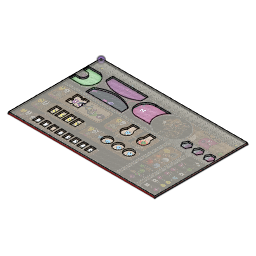
Gaia Project (Autodesk Fusion 360 design; units mm, degrees)
Autodesk Fusion 360 part; units mm, degrees
sketch "Sketch1" plane through (0, 0, 0) normal (0, 1, 0) x (1, 0, 0)
  line L0 (0, 0) -> (300, 0)
  line L1 (300, 0) -> (300, -190)
  line L2 (300, -190) -> (0, -190)
  line L3 (0, -190) -> (0, 0)
  dimension "d1" = 300
  dimension "d2" = 190
  constraint horizontal L0
  constraint vertical L1
  constraint horizontal L2
  constraint vertical L3
  constraint coincident L0.start L3.end
  measures "d1" distance of L0.start L0.end
  measures "d2" distance of L0.start L2.end
sketch "Sketch2" plane through (0, 0, 0) normal (0, 1, 0) x (1, 0, 0)
  line L0 (0, 0) -> (300, 0)
  line L1 (300, 0) -> (300, -190)
  line L2 (300, -190) -> (0, -190)
  line L3 (0, -190) -> (0, 0)
  line L4 (38.8424, -166.0412) -> (48.8424, -166.0412)
  line L5 (48.8424, -166.0412) -> (48.8424, -180.0412)
  line L6 (48.8424, -180.0412) -> (38.8424, -180.0412)
  line L7 (38.8424, -180.0412) -> (38.8424, -166.0412)
  line L8 (64.0567, -180.0412) -> (54.0567, -180.0412)
  line L9 (54.0567, -180.0412) -> (54.0567, -166.0412)
  line L10 (54.0567, -166.0412) -> (64.0567, -166.0412)
  line L11 (64.0567, -166.0412) -> (64.0567, -180.0412)
  line L12 (79.271, -180.0412) -> (69.271, -180.0412)
  line L13 (69.271, -180.0412) -> (69.271, -166.0412)
  line L14 (69.271, -166.0412) -> (79.271, -166.0412)
  line L15 (79.271, -166.0412) -> (79.271, -180.0412)
  line L16 (94.4853, -180.0412) -> (84.4853, -180.0412)
  line L17 (84.4853, -180.0412) -> (84.4853, -166.0412)
  line L18 (84.4853, -166.0412) -> (94.4853, -166.0412)
  line L19 (94.4853, -166.0412) -> (94.4853, -180.0412)
  line L20 (109.6995, -180.0412) -> (99.6995, -180.0412)
  line L21 (99.6995, -180.0412) -> (99.6995, -166.0412)
  line L22 (99.6995, -166.0412) -> (109.6995, -166.0412)
  line L23 (109.6995, -166.0412) -> (109.6995, -180.0412)
  line L24 (124.9138, -180.0412) -> (114.9138, -180.0412)
  line L25 (114.9138, -180.0412) -> (114.9138, -166.0412)
  line L26 (114.9138, -166.0412) -> (124.9138, -166.0412)
  line L27 (124.9138, -166.0412) -> (124.9138, -180.0412)
  line L28 (140.1281, -180.0412) -> (130.1281, -180.0412)
  line L29 (130.1281, -180.0412) -> (130.1281, -166.0412)
  line L30 (130.1281, -166.0412) -> (140.1281, -166.0412)
  line L31 (140.1281, -166.0412) -> (140.1281, -180.0412)
  line L32 (155.3424, -180.0412) -> (145.3424, -180.0412)
  line L33 (145.3424, -180.0412) -> (145.3424, -166.0412)
  line L34 (145.3424, -166.0412) -> (155.3424, -166.0412)
  line L35 (155.3424, -166.0412) -> (155.3424, -180.0412)
  line L36 (38.4602, -129.9646) -> (49.4602, -129.9646)
  line L37 (49.4602, -129.9646) -> (49.4602, -148.9646)
  line L38 (49.4602, -148.9646) -> (38.4602, -148.9646)
  line L39 (38.4602, -148.9646) -> (38.4602, -129.9646)
  line L40 (53.6269, -129.9646) -> (64.6269, -129.9646)
  line L41 (64.6269, -129.9646) -> (64.6269, -148.9646)
  line L42 (64.6269, -148.9646) -> (53.6269, -148.9646)
  line L43 (53.6269, -148.9646) -> (53.6269, -129.9646)
  line L44 (68.7936, -129.9646) -> (79.7936, -129.9646)
  line L45 (79.7936, -129.9646) -> (79.7936, -148.9646)
  line L46 (79.7936, -148.9646) -> (68.7936, -148.9646)
  line L47 (68.7936, -148.9646) -> (68.7936, -129.9646)
  line L48 (83.9602, -129.9646) -> (94.9602, -129.9646)
  line L49 (94.9602, -129.9646) -> (94.9602, -148.9646)
  line L50 (94.9602, -148.9646) -> (83.9602, -148.9646)
  line L51 (83.9602, -148.9646) -> (83.9602, -129.9646)
  circle A0 centre (151.5176, -138.9113) radius 9.55
  circle A1 centre (173.7676, -138.9113) radius 9.55
  circle A2 centre (196.0176, -138.9113) radius 9.55
  line L52 (163.1466, -84.6487) -> (163.1466, -96.6053)
  line L53 (150.1466, -96.8262) -> (150.1466, -84.6487)
  arc A3 (150.1466, -96.8262) -> (163.1466, -96.6053) centre (156.7757, -104.3132) ccw
  line L54 (150.1466, -84.6487) -> (163.1466, -84.6487)
  arc A4 (184.1466, -96.8262) -> (197.1466, -96.6053) centre (190.7757, -104.3132) ccw
  line L55 (184.1466, -96.8262) -> (184.1466, -84.6487)
  line L56 (184.1466, -84.6487) -> (197.1466, -84.6487)
  line L57 (197.1466, -84.6487) -> (197.1466, -96.6053)
  line L58 (39.1516, -88.1384) -> (49.1516, -88.1384)
  line L59 (49.1516, -88.1384) -> (49.1516, -90.2914)
  line L60 (41.8914, -98.1384) -> (39.1516, -98.1384)
  line L61 (39.1516, -98.1384) -> (39.1516, -88.1384)
  line L62 (39.1516, -102.1384) -> (41.8914, -102.1384)
  line L63 (49.1516, -110.2914) -> (49.1516, -112.1384)
  line L64 (49.1516, -112.1384) -> (39.1516, -112.1384)
  line L65 (39.1516, -112.1384) -> (39.1516, -102.1384)
  line L66 (64.1516, -98.1384) -> (61.8914, -98.1384)
  line L67 (54.1516, -90.2914) -> (54.1516, -88.1384)
  line L68 (54.1516, -88.1384) -> (64.1516, -88.1384)
  line L69 (64.1516, -88.1384) -> (64.1516, -98.1384)
  line L70 (64.1516, -112.1384) -> (54.1516, -112.1384)
  line L71 (54.1516, -112.1384) -> (54.1516, -110.2914)
  line L72 (64.1516, -102.1384) -> (64.1516, -112.1384)
  line L73 (61.8914, -102.1384) -> (64.1516, -102.1384)
  line L74 (49.1516, -90.2914) -> (54.1516, -90.2914)
  line L75 (54.1516, -110.2914) -> (49.1516, -110.2914)
  line L76 (41.8914, -102.1384) -> (41.8914, -98.1384)
  line L77 (61.8914, -98.1384) -> (61.8914, -102.1384)
  line L78 (43.9458, -20.2003) -> (116.6031, -20.2003)
  line L79 (116.6031, -20.2003) -> (116.6031, -32.6832)
  line L80 (43.9458, -32.6832) -> (43.9458, -20.2003)
  arc A5 (45.5061, -35.5966) -> (115.0427, -35.5966) centre (80.2744, 16.6243) ccw
  arc A6 (43.9458, -32.6832) -> (45.5061, -35.5966) centre (47.4458, -32.6832) ccw
  arc A7 (115.0427, -35.5966) -> (116.6031, -32.6832) centre (113.1031, -32.6832) ccw
  line L81 (43.6031, -74.6832) -> (43.6031, -62.2003)
  line L82 (116.2603, -74.6832) -> (43.6031, -74.6832)
  line L83 (116.2603, -62.2003) -> (116.2603, -74.6832)
  arc A8 (116.2603, -62.2003) -> (114.7, -59.2869) centre (112.7603, -62.2003) ccw
  arc A9 (114.7, -59.2869) -> (45.1634, -59.2869) centre (79.9317, -111.5078) ccw
  arc A10 (45.1634, -59.2869) -> (43.6031, -62.2003) centre (47.1031, -62.2003) ccw
  line L84 (138.2548, -26.8165) -> (169.9814, -26.8165)
  line L85 (166.6088, -66.8165) -> (138.2548, -66.8165)
  line L86 (138.2548, -66.8165) -> (138.2548, -66.8115)
  arc A11 (169.9814, -26.8165) -> (166.6088, -66.8165) centre (187.3421, -48.4225) ccw
  arc A12 (138.8864, -26.8165) -> (138.2548, -66.8115) centre (138.5706, -46.814) ccw
  line L87 (250.9752, -65.9327) -> (246.3444, -57.9397)
  line L88 (246.3444, -57.9397) -> (237.1068, -57.9536)
  line L89 (237.1068, -57.9536) -> (232.5, -65.9606)
  line L90 (232.5, -65.9606) -> (237.1309, -73.9536)
  line L91 (237.1309, -73.9536) -> (246.3685, -73.9397)
  line L92 (246.3685, -73.9397) -> (250.9752, -65.9327)
  line L93 (237.1068, -57.9536) -> (232.5, -65.9606)
  line L94 (232.5, -65.9606) -> (237.1309, -73.9536)
  line L95 (237.1309, -73.9536) -> (246.3685, -73.9397)
  line L96 (246.3685, -73.9397) -> (250.9752, -65.9327)
  line L97 (250.9752, -65.9327) -> (246.3444, -57.9397)
  line L98 (246.3444, -57.9397) -> (237.1068, -57.9536)
  line L99 (237.1068, -57.9536) -> (232.5, -65.9606)
  line L100 (232.5, -65.9606) -> (237.1309, -73.9536)
  line L101 (237.1309, -73.9536) -> (246.3685, -73.9397)
  line L102 (246.3685, -73.9397) -> (250.9752, -65.9327)
  line L103 (246.3444, -57.9397) -> (237.1068, -57.9536)
  line L104 (250.9752, -65.9327) -> (246.3444, -57.9397)
  line L105 (260.3568, -57.9536) -> (255.75, -65.9606)
  line L106 (255.75, -65.9606) -> (260.3809, -73.9536)
  line L107 (260.3809, -73.9536) -> (269.6185, -73.9397)
  line L108 (269.6185, -73.9397) -> (274.2252, -65.9327)
  line L109 (274.2252, -65.9327) -> (269.5944, -57.9397)
  line L110 (269.5944, -57.9397) -> (260.3568, -57.9536)
  line L111 (283.6068, -57.9536) -> (279, -65.9606)
  line L112 (279, -65.9606) -> (283.6309, -73.9536)
  line L113 (283.6309, -73.9536) -> (292.8685, -73.9397)
  line L114 (292.8685, -73.9397) -> (297.4752, -65.9327)
  line L115 (297.4752, -65.9327) -> (292.8444, -57.9397)
  line L116 (292.8444, -57.9397) -> (283.6068, -57.9536)
  line L117 (1.8268, -27.4135) -> (26.074, -27.4135)
  line L118 (26.074, -67.4135) -> (1.8268, -67.4135)
  arc A13 (26.074, -67.4135) -> (26.074, -27.4135) centre (19.5792, -47.4135) ccw
  line L119 (1.8268, -38.5158) -> (11.1453, -38.5158)
  line L120 (11.0214, -55.1916) -> (1.8268, -55.1916)
  arc A14 (11.0214, -55.1916) -> (11.1453, -38.5158) centre (9.4323, -46.8414) ccw
  line L121 (1.8268, -67.4135) -> (1.8268, -55.1916)
  line L122 (1.8268, -38.5158) -> (1.8268, -27.4135)
  point P0 (241.7376, -65.9467)
  dimension "d3" = 300
  dimension "d4" = 190
  dimension "d5" = 10
  dimension "d6" = 14
  dimension "d9" = 106.5
  dimension "d10" = 0
  dimension "d11" = 11
  dimension "d12" = 19
  dimension "d15" = 45.5
  dimension "d16" = 0
  dimension "d17" = 19.1
  dimension "d20" = 44.5
  dimension "d21" = 0
  dimension "d22" = 20
  dimension "d23" = 13
  dimension "d24" = 20
  dimension "d25" = 13
  dimension "d26" = 10
  dimension "d27" = 10
  dimension "d29" = 10
  dimension "d30" = 10
  dimension "d36" = 3.5
  dimension "d37" = 3.5
  dimension "d38" = 40
  dimension "d40" = 40
  dimension "d41" = 8
  dimension "d44" = 46.5
  dimension "d45" = 0
  dimension "d46" = 17
  dimension "d47" = 24.2472
  dimension "d48" = 40
  constraint horizontal L0
  constraint vertical L1
  constraint horizontal L2
  constraint vertical L3
  constraint coincident L0.start L3.end
  constraint horizontal L4
  constraint vertical L5
  constraint horizontal L6
  constraint vertical L7
  constraint horizontal L36
  constraint vertical L37
  constraint horizontal L38
  constraint vertical L39
  constraint vertical L52
  constraint vertical L53
  constraint perpendicular L52 L54
  constraint vertical L57
  constraint vertical L55
  constraint perpendicular L56 L57
  constraint horizontal L58
  constraint vertical L59
  constraint horizontal L60
  constraint vertical L61
  constraint horizontal L62
  constraint vertical L63
  constraint horizontal L64
  constraint vertical L65
  constraint horizontal L68
  constraint vertical L69
  constraint horizontal L66
  constraint vertical L67
  constraint horizontal L73
  constraint vertical L72
  constraint horizontal L70
  constraint vertical L71
  constraint horizontal L74
  constraint horizontal L75
  constraint vertical L76
  constraint perpendicular L73 L77
  constraint horizontal L78
  constraint vertical L79
  constraint vertical L80
  constraint tangent L80 A6
  constraint tangent A5 A6
  constraint tangent A5 A7
  constraint tangent L79 A7
  constraint equal A6 A7
  constraint tangent L83 A8
  constraint tangent A8 A9
  constraint tangent A9 A10
  constraint tangent L81 A10
  constraint equal A8 A10
  constraint horizontal L84
  constraint horizontal L85
  constraint vertical L86
  constraint coincident L84.start A12
  constraint coincident L84 A12.start
  constraint horizontal L117
  constraint horizontal L118
  constraint vertical L121
  constraint horizontal L119
  constraint horizontal L120
  constraint coincident L119.start L121
  constraint collinear L121 L122
  measures "d3" distance of L0.start L0.end
  measures "d4" distance of L0.start L2.end
  measures "d5" distance of L4.start L4.end
  measures "d6" distance of L4.start L6.end
  measures "d11" distance of L36.start L36.end
  measures "d12" distance of L36.start L38.end
  measures "d17" diameter of A0
  measures "d22" diameter of A3
  measures "d23" distance of L53.end L52.start
  measures "d24" diameter of A4
  measures "d25" distance of L55.end L56.end
  measures "d26" distance of L58.start L58.end
  measures "d27" distance of L58.start L60.end
  measures "d29" distance of L64.end L62.start
  measures "d30" distance of L68.end L67.end
  measures "d36" radius of A6
  measures "d37" radius of A8
  measures "d38" diameter of A12
  measures "d40" distance of L84.start L85.end
  measures "d41" distance of P0 L92
  measures "d46" diameter of A14
  measures "d47" distance of L117.start L117.end
  measures "d48" distance of L117.start L118.end
extrude "Extrude1" add sketch "Sketch2" along normal blind 3
